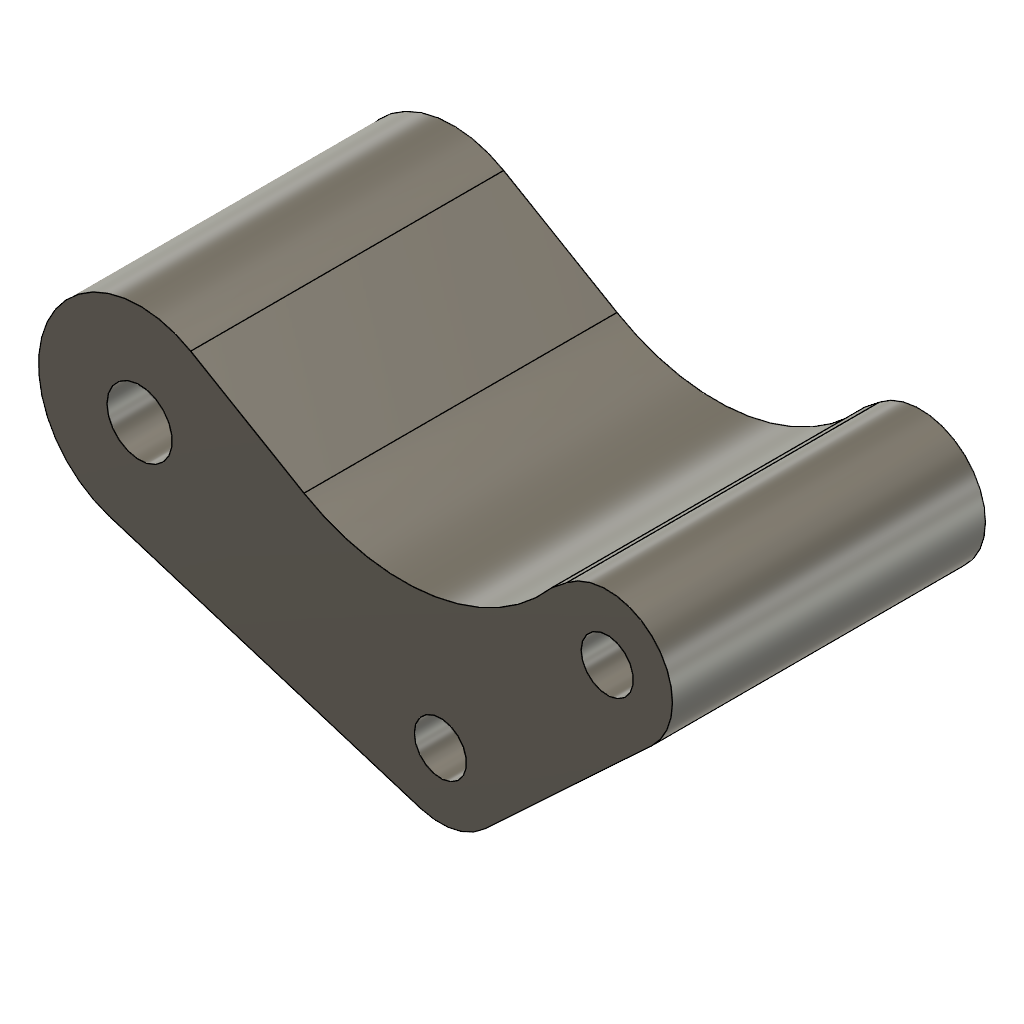
Bracket-PZ (Autodesk Fusion 360 design; units mm, degrees)
Autodesk Fusion 360 part; units mm, degrees
sketch "Sketch1" plane through (0, 0, 0) normal (0, 0, 1) x (1, 0, 0)
  circle A0 centre (0, 0) radius 15.5
  circle A1 centre (71.699, 3.628) radius 10
  line L0 (-4.625, -14.7939) -> (43.1361, -29.7254)
  line L1 (52.9333, -27.5008) -> (78.5123, -3.6918)
  arc A2 (43.1361, -29.7254) -> (52.9333, -27.5008) centre (46.12, -20.181) ccw
  line L2 (7.8289, 13.3775) -> (25.2043, 3.209)
  arc A3 (25.2043, 3.209) -> (63.1836, 9.6345) centre (40.357, 29.101) ccw
  line L3 (63.1836, 9.6345) -> (65.4783, 11.4576)
  dimension "d1" = 10
  dimension "d2" = 31
  dimension "d3" = 20
  dimension "d4" = 3.628
  dimension "d5" = 71.699
  dimension "d6" = 40.357
  dimension "d7" = 30
  dimension "d9" = 20.181
  dimension "d10" = 46.12
  dimension "d12" = 29.101
  constraint coincident A0.centre origin
  constraint coincident A0 L0.start
  constraint tangent A0 L0
  constraint coincident A1 L1.end
  constraint tangent A1 L1
  constraint tangent L0 A2
  constraint tangent L1 A2
  constraint coincident A0 L2.start
  constraint tangent A0 L2
  constraint tangent L2 A3
  constraint coincident A1 L3.end
  constraint tangent A1 L3
  measures "d1" radius of A2
  measures "d2" diameter of A0
  measures "d3" diameter of A1
  measures "d4" vertical distance of A0.centre A1.centre
  measures "d5" horizontal distance of A0.centre A1.centre
  measures "d6" horizontal distance of A0.centre A3.centre
  measures "d7" radius of A3
  measures "d9" vertical distance of A0.centre A2.centre
  measures "d10" horizontal distance of A0.centre A2.centre
  measures "d12" vertical distance of A0.centre A3.centre
extrude "Extrude1" add sketch "Sketch1" along normal blind 48
sketch "Sketch2" plane through (0, 0, 48) normal (0, 0, 1) x (1, 0, 0)
  arc A0 (7.8289, 13.3775) -> (-4.625, -14.7939) centre (0, 0) ccw
  line L0 (-4.625, -14.7939) -> (43.1361, -29.7254)
  arc A1 (43.1361, -29.7254) -> (52.9333, -27.5008) centre (46.12, -20.181) ccw
  line L1 (52.9333, -27.5008) -> (78.5123, -3.6918)
  arc A2 (78.5123, -3.6918) -> (65.4783, 11.4576) centre (71.699, 3.628) ccw
  line L2 (65.4783, 11.4576) -> (63.1836, 9.6345)
  arc A3 (25.2043, 3.209) -> (63.1836, 9.6345) centre (40.357, 29.101) ccw
  line L3 (25.2043, 3.209) -> (7.8289, 13.3775)
  circle A4 centre (0, 0) radius 5
  circle A5 centre (46.12, -20.181) radius 4
  circle A6 centre (71.699, 3.628) radius 4
  dimension "d19" = 8
  dimension "d20" = 8
  constraint concentric A0 A4
  constraint concentric A1 A5
  constraint concentric A2 A6
  measures "d19" diameter of A5
  measures "d20" diameter of A6
extrude "Extrude2" cut sketch "Sketch2" against normal blind 48 contours A4 | A5 | A6
